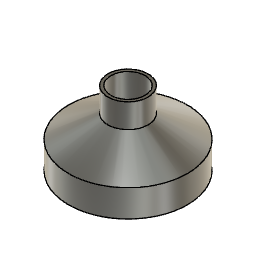
buje (Autodesk Fusion 360 design; units mm, degrees)
Autodesk Fusion 360 part; units mm, degrees
sketch "Boceto1" plane through (0, 0, 0) normal (0, 0, 1) x (1, 0, 0)
  circle A0 centre (0, 0) radius 39.5
  circle A1 centre (0, 0) radius 36
  dimension "d1" = 79
  dimension "d2" = -3.5
  constraint coincident A0.centre A1.centre
  measures "d1" diameter of A0
ref_plane "PlanoDeObra1" through (0, 0, 15) normal (0, 0, 1) x (1, 0, 0)
sketch "Boceto2" plane through (0, 0, 15) normal (0, 0, 1) x (1, 0, 0)
  circle A0 centre (0, 0) radius 13.375
  circle A1 centre (0, 0) radius 11.375
  dimension "d4" = 26.75
  dimension "d5" = -2
  constraint coincident A0.centre A1.centre
  measures "d4" diameter of A0
loft "Solevación1" add profiles "Boceto1", "Boceto2" section 1 section 2
loft "Solevación2" cut profiles "Boceto2", "Boceto1" section 1 contours A1 section 2 contours A1
extrude "Extruir1" add sketch "Boceto2" along normal blind 16
extrude "Extruir2" add sketch "Boceto1" against normal blind 18
